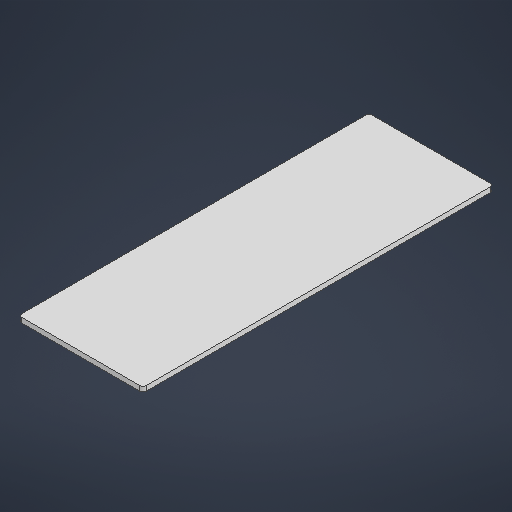
# Autodesk Inventor part: module-lid_command
Saved by Autodesk Inventor 2025.2 (Build 292293000, 293)
## iProperties
Created: 2025-09-05
Part Number: module-lid_command
Material: Generic
Document SubType Name: Modeling
Designer: sam
Density: 1 g/cm^3
Appearance: Default
Author: sam
Autodesk Inventor part; units mm, degrees
ref_plane "YZ Plane" through (0, 0, 0) normal (1, 0, 0) x (0, 1, 0)
ref_plane "XZ Plane" through (0, 0, 0) normal (0, 1, 0) x (-1, 0, 0)
ref_plane "XY Plane" through (0, 0, 0) normal (0, 0, 1) x (1, 0, 0)
sketch "Sketch1" plane through (0, 0, 0) normal (0, 1, 0) x (-1, 0, 0)
  line L0 (-38, -107) -> (38, -107)
  line L1 (38, -107) -> (38, 107)
  line L2 (38, 107) -> (-38, 107)
  line L3 (-38, 107) -> (-38, -107)
  line L4 (-38, -107) -> (38, 107) construction
  line L5 (38, -107) -> (-38, 107) construction
  point P0 (0, 0)
  dimension "d0" = 76
  dimension "d1" = 214
  constraints: 12 end point, 2 midpoint, 2 parallel, 1 horizontal, 1 perpendicular
  measures "d0" distance of L2.end L1.end
  measures "d1" distance of L1.end L0.end
extrude "Extrusion1" add sketch "Sketch1" against normal blind 3
sketch "Sketch2" plane through (0, -3, 0) normal (0, -1, 0) x (1, 0, 0)
  line L0 (-38, 107) -> (-38, -107) projected
  line L1 (-38, -107) -> (38, -107) projected
  line L2 (38, -107) -> (38, 107) projected
  line L3 (38, 107) -> (-38, 107) projected
  line L4 (35, 104) -> (-35, 104)
  line L5 (-35, 104) -> (-35, -104)
  line L6 (-35, -104) -> (35, -104)
  line L7 (35, -104) -> (35, 104)
  line L8 (35, 104) -> (-35, -104) construction
  line L9 (-35, 104) -> (35, -104) construction
  point P0 (0, 0)
  dimension "d4" = 3
  dimension "d5" = 3
  constraints: 12 end point, 2 midpoint, 2 parallel, 1 horizontal, 1 perpendicular
  measures "d4" distance between parallel lines of L5 L0
  measures "d5" distance between parallel lines of L1 L6
extrude "Extrusion2" add sketch "Sketch2" along normal blind 3 contours L7 L6 L5 L4
fillet "Fillet1" radius 2 8 edges at (35, -4.5, 104) (-35, -4.5, 104) (38, -1.5, 107) (-38, -1.5, 107) (35, -4.5, -104) (38, -1.5, -107) (-35, -4.5, -104) (-38, -1.5, -107)
body "Solid1"
